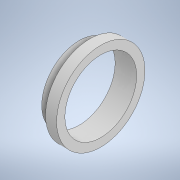
# Autodesk Inventor part: 轴套2
Saved by Autodesk Inventor 2020 (Build 240168000, 168)
## iProperties
Created: 2021-06-17
Part Number: 轴套2
Material: 常规
Document SubType Name: Modeling
Designer: dell
Density: 1 g/cm^3
Appearance: 默认
Author: dell
Autodesk Inventor part; units mm, degrees
ref_plane "YZ Plane" through (0, 0, 0) normal (1, 0, 0) x (0, 1, 0)
ref_plane "XZ Plane" through (0, 0, 0) normal (0, 1, 0) x (-1, 0, 0)
ref_plane "XY Plane" through (0, 0, 0) normal (0, 0, 1) x (1, 0, 0)
sketch "草图1" plane through (0, 0, 0) normal (0, 0, 1) x (1, 0, 0)
  line L0 (-23.4, 0) -> (3.9, 0) construction
  line L1 (0, -56) -> (0, 56) construction
  line L2 (-19.5, 34) -> (-10, 34)
  line L3 (-10, -34) -> (-19.5, -34)
  line L4 (-19.5, -34) -> (-19.5, 34)
  line L5 (-10, 40) -> (0, 40)
  line L6 (0, 40) -> (0, -40)
  line L7 (0, -40) -> (-10, -40)
  line L8 (-10, -40) -> (-10, -34)
  line L9 (-10, 34) -> (-10, 40)
  line L10 (-19.5, 32.5) -> (0, 32.5)
  line L11 (0, 32.5) -> (0, -32.5)
  line L12 (0, -32.5) -> (-19.5, -32.5)
  line L13 (-19.5, -32.5) -> (-19.5, 32.5)
  point P0 (0, 0)
  point P1 (0, 32.5)
  dimension "d0" = 68
  dimension "d1" = 65
  dimension "d2" = 19.5
  dimension "d3" = 10
  dimension "d4" = 80
  constraints: 24 end point, 6 parallel, 3 horizontal, 2 perpendicular, 2 point on line, 1 collinear, 1 midpoint, 2 other
  measures "d0" distance between parallel lines of L3 L2
  measures "d1" distance between parallel lines of L12 L10
  measures "d2" distance between parallel lines of L11 L13
  measures "d3" distance between parallel lines of L6 L9
  measures "d4" distance between parallel lines of L7 L5
revolve "旋转1" add sketch "草图1" angle 360 about axis through (-10, 0, 0) along (1, 0, 0) contours L2 L9 L5 L6 L10 L4
